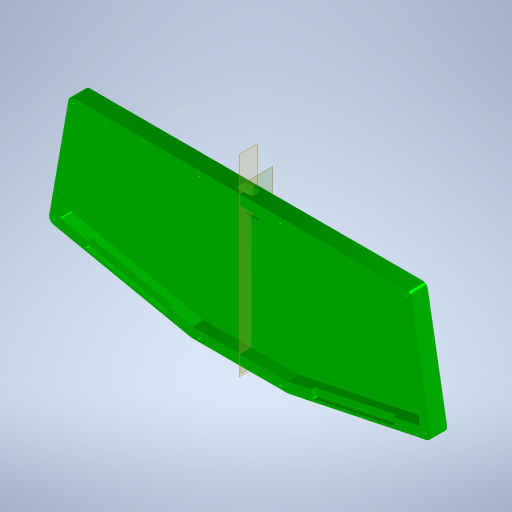
# Autodesk Inventor part: bottom-case
Saved by Autodesk Inventor 2023 (Build 270158000, 158)
## iProperties
Created: 2022-09-09
Part Number: bottom-case
Material: Aluminum 6061-AHC
Document SubType Name: Modeling
Designer: hainguyen
Density: 2.7 g/cm^3
Appearance: Aluminum - Dark
Author: hainguyen
Autodesk Inventor part; units mm, degrees
ref_plane "YZ Plane" through (0, 0, 0) normal (1, 0, 0) x (0, 1, 0)
ref_plane "XZ Plane" through (0, 0, 0) normal (0, 1, 0) x (-1, 0, 0)
ref_plane "XY Plane" through (0, 0, 0) normal (0, 0, 1) x (1, 0, 0)
sketch "Sketch1" plane through (0, 0, 0) normal (0, 0, 1) x (1, 0, 0)
  line L0 (21.6076, -129.4029) -> (96.5033, -129.4029) construction
  line L1 (96.5033, -129.4029) -> (135.6521, -121.1948) construction
  line L2 (-17.5411, -121.1947) -> (21.6076, -129.4029) construction
  line L3 (-68.8789, -30.3383) -> (-82.3292, -106.6218) construction
  line L4 (200.4404, -106.6223) -> (186.9912, -30.3383) construction
  line L5 (121.8455, -29.5119) -> (-68.8789, -29.5119) construction
  line L6 (-69.5723, -28.5119) -> (187.6846, -28.5119)
  line L7 (187.6846, -28.5119) -> (201.7615, -108.3559)
  line L8 (201.7615, -108.3559) -> (96.607, -130.4029)
  line L9 (96.607, -130.4029) -> (21.5039, -130.4029)
  line L10 (21.5039, -130.4029) -> (-83.6503, -108.3555)
  line L11 (-83.6503, -108.3555) -> (-69.5723, -28.5119)
  point P0 (0, 0)
  dimension "d0" = 1
  dimension "d1" = 1
  dimension "d2" = 1
  dimension "d3" = 1
  dimension "d4" = 1
  dimension "d5" = 1
  constraints: 14 end point, 7 parallel, 2 horizontal, 2 other
  measures "d0" distance between parallel lines of L6 L5
  measures "d1" distance between parallel lines of L3 L11
  measures "d2" distance between parallel lines of L2 L10
  measures "d3" distance between parallel lines of L0 L9
  measures "d4" distance between parallel lines of L1 L8
  measures "d5" distance between parallel lines of L4 L7
extrude "Extrusion1" add sketch "Sketch1" along normal blind 17
shell "Shell1" thickness 8 outward yes removed faces 1 at (71.5731, -62.4756, 17)
sketch "Sketch5" plane through (-69.5723, -28.5119, 0) normal (0, 0, 1) x (1, 0, 0)
  line L0 (-14.0781, -79.8436) -> (91.0762, -101.891) projected
  line L1 (91.0762, -101.891) -> (166.1793, -101.891) projected
  line L2 (166.1793, -101.891) -> (271.3337, -79.844) projected
  line L3 (271.3337, -79.844) -> (257.2569, 0) projected
  line L4 (257.2569, 0) -> (0, 0) projected
  line L5 (0, 0) -> (-14.0781, -79.8436) projected
  point P0 (69.5723, 28.5119)
extrude "Extrusion7" add sketch "Sketch5" along normal blind 8
ref_plane "Work Plane1" through (59.0626, 747.1099, -8) normal (-1, 0.0000081, 0) x (0, 0, 1)
sketch "Sketch7" plane through (-76.2851, -20.5119, 17) normal (0, 1, 0) x (1, 0, 0)
  line L0 (131.2466, 4.8) -> (139.4466, 4.8) construction
  line L1 (132.1766, 8.53) -> (138.5266, 8.53) construction
  line L2 (141.8266, 2.8) -> (128.8766, 2.8)
  line L3 (128.8766, 2.8) -> (128.8766, 10.53)
  line L4 (128.8766, 10.53) -> (141.8266, 10.53)
  line L5 (141.8266, 10.53) -> (141.8266, 2.8)
  line L6 (130.8766, 6.67) -> (130.8766, 7.23) construction
  line L7 (139.8266, 7.23) -> (139.8266, 6.67) construction
  point P0 (76.2851, 17)
  point P1 (128.8766, 6.665)
  point P2 (130.8766, 6.95)
  dimension "d25" = 2
  dimension "d26" = 2
  dimension "d27" = 2
  dimension "d28" = 2
  constraints: 8 end point, 2 midpoint, 2 parallel, 1 horizontal, 1 perpendicular
  measures "d25" horizontal distance of point (128.877, 6.665) point (130.877, 6.95)
  measures "d26" distance from line of L5 L7.end
  measures "d27" distance between parallel lines of L1 L4
  measures "d28" distance between parallel lines of L0 L2
extrude "Extrusion9" cut sketch "Sketch7" against normal blind 20
fillet "Fillet2" radius 3 4 edges at (65.5415, -24.5119, 14.2) (65.5415, -30.5119, 6.47) (52.5915, -24.5119, 14.2) (52.5915, -30.5119, 6.47)
sketch "Sketch12" plane through (0, 0, 17) normal (0, 0, 1) x (1, 0, 0)
  line L0 (102.8455, -23.0119) -> (165.8455, -23.0119) construction
  line L1 (121.8455, -29.5119) -> (-67.894, -29.5119) construction
  line L2 (121.8455, -29.5119) -> (-67.894, -29.5119) construction
  line L3 (-47.7327, -23.0102) -> (15.2673, -23.0112) construction
  line L4 (-17.5411, -121.1947) -> (21.6076, -129.4029) construction
  line L5 (-0.2792, -131.4544) -> (-61.9383, -118.5257) construction
  line L6 (180.0496, -118.5277) -> (118.3902, -131.4553) construction
  line L7 (96.5033, -129.4029) -> (135.6521, -121.1948) construction
  line L8 (167.3455, -29.5119) -> (167.3455, -22.5119)
  line L9 (167.3455, -22.5119) -> (101.3455, -22.5119)
  line L10 (101.3455, -22.5119) -> (101.3455, -29.5119)
  line L11 (101.3455, -29.5119) -> (167.3455, -29.5119)
  line L12 (16.7672, -29.5119) -> (16.7672, -22.5119)
  line L13 (16.7672, -22.5119) -> (-49.2328, -22.5119)
  line L14 (16.7672, -29.5119) -> (-49.2328, -29.5119)
  line L15 (96.5033, -129.4029) -> (135.6521, -121.1948) construction
  line L16 (115.5884, -125.4015) -> (117.0248, -132.2525)
  line L17 (117.0248, -132.2525) -> (181.6203, -118.7092)
  line L18 (181.6203, -118.7092) -> (180.1839, -111.8582)
  line L19 (115.5884, -125.4015) -> (180.1839, -111.8582)
  line L20 (-81.5496, -107.7742) -> (-42.0091, -116.0645) construction
  line L21 (2.5226, -125.4014) -> (1.0863, -132.2516)
  line L22 (-63.509, -118.7073) -> (-62.0728, -111.8578)
  line L23 (2.5226, -125.4014) -> (-62.0728, -111.8578)
  line L24 (1.0863, -132.2516) -> (-63.509, -118.7073)
  line L25 (-42.4192, -118.0206) -> (-42.0091, -116.0645) construction
  line L26 (-17.5411, -121.1947) -> (-17.9513, -123.151) construction
  line L27 (136.0625, -123.1523) -> (135.6521, -121.1948) construction
  line L28 (121.8455, -29.5119) -> (121.8455, -27.5119) construction
  line L29 (-3.7328, -27.5109) -> (-3.7328, -29.5109) construction
  line L30 (-28.7328, -29.5105) -> (-28.7328, -27.5105) construction
  line L31 (-49.2328, -22.5119) -> (-49.2328, -29.5119)
  line L32 (160.5305, -118.0223) -> (160.1201, -116.0648) construction
  line L33 (146.8455, -29.5119) -> (146.8455, -27.5119) construction
  point P0 (-49.2327, -26.0119)
  point P1 (-28.7328, -28.5105)
  dimension "d48" = 0.5
  dimension "d50" = 0.5
  dimension "d51" = 20.5
  dimension "d52" = 20.5
  dimension "d53" = 20.5
  dimension "d56" = 0.5
  dimension "d57" = 20.5
  dimension "d58" = 20.5
  dimension "d60" = 20.5
  dimension "d78" = 20.5
  dimension "d80" = 20.5
  constraints: 32 end point, 10 point on line, 7 perpendicular, 3 collinear, 3 parallel, 2 vertical, 1 midpoint
  measures "d48" distance between parallel lines of L17 L6
  measures "d50" distance between parallel lines of L24 L5
  measures "d51" distance between parallel lines of L22 L25
  measures "d52" distance between parallel lines of L21 L26
  measures "d53" distance between parallel lines of L16 L27
  measures "d56" distance between parallel lines of L9 L0
  measures "d57" distance between parallel lines of L10 L28
  measures "d58" distance from line of L29.start L12
  measures "d60" distance from line of L31 point (-28.733, -28.51)
  measures "d78" distance between parallel lines of L18 L32
  measures "d80" distance between parallel lines of L8 L33
extrude "Extrusion13" cut sketch "Sketch12" against normal blind 3
fillet "Fillet4" radius 4 4 edges at (-76.2851, -20.5119, 4.5) (194.3976, -20.5119, 4.5) (210.985, -114.5961, 4.5) (-92.874, -114.5955, 4.5)
fillet "Fillet5" radius 1 12 edges at (101.3455, -22.5119, 15.5) (167.3455, -22.5119, 15.5) (187.6846, -28.5119, 12.5) (-49.2328, -22.5119, 15.5) (16.7672, -22.5119, 15.5) (181.6203, -118.7092, 15.5) (117.0248, -132.2525, 15.5) (1.0863, -132.2516, 15.5) (-63.509, -118.7073, 15.5) (-69.5723, -28.5119, 12.5) (-83.6503, -108.3555, 12.5) (201.7615, -108.3559, 12.5)
sketch "Sketch14" plane through (0, 0, -8) normal (0, 0, -1) x (-1, 0, 0)
  arc A0 (89.083, -115.3904) -> (92.2014, -110.7809) centre (88.2622, -111.4755) ccw projected
  line L0 (76.8679, -23.8173) -> (92.2014, -110.7809) projected
  arc A1 (76.8679, -23.8173) -> (72.9287, -20.5119) centre (72.9287, -24.5119) ccw projected
  line L1 (-191.0411, -20.5119) -> (72.9287, -20.5119) projected
  arc A2 (-191.0411, -20.5119) -> (-194.9804, -23.8174) centre (-191.0411, -24.5119) ccw projected
  line L2 (-210.3125, -110.7815) -> (-194.9804, -23.8174) projected
  arc A3 (-210.3125, -110.7815) -> (-207.194, -115.3909) centre (-206.3732, -111.476) ccw projected
  line L3 (-97.4367, -138.4029) -> (-207.194, -115.3909) projected
  line L4 (-20.6743, -138.4029) -> (-97.4367, -138.4029) projected
  line L5 (89.083, -115.3904) -> (-20.6743, -138.4029) projected
  point P0 (0, 0)
extrude "Extrusion14" cut sketch "Sketch14" against normal blind 12
sketch "Sketch16" plane through (0, 0, 4) normal (0, 0, -1) x (-1, 0, 0)
  point P0 (0, 0)
sketch "Sketch17" plane through (0, 0, 4) normal (0, 0, -1) x (-1, 0, 0)
  arc A0 (89.083, -115.3904) -> (92.2014, -110.7809) centre (88.2622, -111.4755) ccw projected
  line L0 (89.083, -115.3904) -> (-20.6743, -138.4029) projected
  line L1 (-20.6743, -138.4029) -> (-97.4367, -138.4029) projected
  line L2 (-97.4367, -138.4029) -> (-207.194, -115.3909) projected
  arc A1 (-210.3125, -110.7815) -> (-207.194, -115.3909) centre (-206.3732, -111.476) ccw projected
  line L3 (-210.3125, -110.7815) -> (-194.9804, -23.8174) projected
  arc A2 (-191.0411, -20.5119) -> (-194.9804, -23.8174) centre (-191.0411, -24.5119) ccw projected
  line L4 (-191.0411, -20.5119) -> (72.9287, -20.5119) projected
  arc A3 (76.8679, -23.8173) -> (72.9287, -20.5119) centre (72.9287, -24.5119) ccw projected
  line L5 (76.8679, -23.8173) -> (92.2014, -110.7809) projected
  line L6 (-2.3174, -126.3801) -> (-1.2915, -131.2729) projected
  arc A4 (-1.2915, -131.2729) -> (-0.1076, -132.0464) centre (-0.3128, -131.0676) ccw projected
  line L7 (-0.1076, -132.0464) -> (62.5303, -118.9125) projected
  arc A5 (62.5303, -118.9125) -> (63.3038, -117.7286) centre (62.3251, -117.9338) ccw projected
  line L8 (63.3038, -117.7286) -> (62.278, -112.8365) projected
  line L9 (62.278, -112.8365) -> (82.7026, -108.5542) projected
  arc A6 (82.7026, -108.5542) -> (83.4822, -107.4018) centre (82.4974, -107.5755) ccw projected
  line L10 (83.4822, -107.4018) -> (69.718, -29.3383) projected
  arc A7 (69.718, -29.3383) -> (68.7332, -28.5119) centre (68.7332, -29.5119) ccw projected
  line L11 (68.7332, -28.5119) -> (49.2328, -28.5119) projected
  line L12 (49.2328, -28.5119) -> (49.2328, -23.5119) projected
  arc A8 (49.2328, -23.5119) -> (48.2328, -22.5119) centre (48.2328, -23.5119) ccw projected
  line L13 (48.2328, -22.5119) -> (-15.7672, -22.5119) projected
  arc A9 (-15.7672, -22.5119) -> (-16.7672, -23.5119) centre (-15.7672, -23.5119) ccw projected
  line L14 (-16.7672, -23.5119) -> (-16.7672, -28.5119) projected
  line L15 (-16.7672, -28.5119) -> (-101.3455, -28.5119) projected
  line L16 (-101.3455, -28.5119) -> (-101.3455, -23.5119) projected
  arc A10 (-101.3455, -23.5119) -> (-102.3455, -22.5119) centre (-102.3455, -23.5119) ccw projected
  line L17 (-102.3455, -22.5119) -> (-166.3455, -22.5119) projected
  arc A11 (-166.3455, -22.5119) -> (-167.3455, -23.5119) centre (-166.3455, -23.5119) ccw projected
  line L18 (-167.3455, -23.5119) -> (-167.3455, -28.5119) projected
  line L19 (-167.3455, -28.5119) -> (-186.8455, -28.5119) projected
  arc A12 (-186.8455, -28.5119) -> (-187.8303, -29.3383) centre (-186.8455, -29.5119) ccw projected
  line L20 (-187.8303, -29.3383) -> (-201.5933, -107.4023) projected
  arc A13 (-201.5933, -107.4023) -> (-200.8137, -108.5546) centre (-200.6085, -107.5759) ccw projected
  line L21 (-200.8137, -108.5546) -> (-180.3891, -112.8369) projected
  line L22 (-180.3891, -112.8369) -> (-181.4151, -117.7305) projected
  arc A14 (-181.4151, -117.7305) -> (-180.6416, -118.9145) centre (-180.4364, -117.9357) ccw projected
  line L23 (-180.6416, -118.9145) -> (-118.0035, -132.0473) projected
  arc A15 (-118.0035, -132.0473) -> (-116.8196, -131.2738) centre (-117.7983, -131.0686) ccw projected
  line L24 (-116.8196, -131.2738) -> (-115.7936, -126.3802) projected
  line L25 (-115.7936, -126.3802) -> (-96.607, -130.4029) projected
  line L26 (-96.607, -130.4029) -> (-21.5039, -130.4029) projected
  line L27 (-21.5039, -130.4029) -> (-2.3174, -126.3801) projected
  circle A16 centre (-191.0411, -24.5119) radius 1.7396
  circle A17 centre (-206.3732, -111.476) radius 1.3455
  circle A18 centre (-91.1144, -135.6415) radius 1.736
  circle A19 centre (-91.1144, -24.5119) radius 2.0059
  line L28 (-91.1144, -24.5119) -> (-91.1144, -135.6415)
  line L29 (-91.1144, -135.6415) -> (-206.3732, -111.476) construction
  line L30 (-191.0411, -24.5119) -> (-91.1144, -24.5119) construction
  line L31 (-191.0411, -24.5119) -> (-206.3732, -111.476) construction
  line L32 (-59.0568, 27.6823) -> (-59.0553, -166.0852) projected
  circle A20 centre (72.9283, -24.5098) radius 1.7396
  circle A21 centre (88.2618, -111.4736) radius 1.3455
  circle A22 centre (-26.9966, -135.6409) radius 1.736
  circle A23 centre (-26.9984, -24.5114) radius 2.0059
  point P0 (0, 0)
  dimension "d83" = 64.116
  constraints: 8 centre point, 8 end point, 4 symmetric about line, 2 coincident, 2 parallel, 1 vertical, 4 other
  measures "d83" distance of A23.centre L28.start
ref_plane "Work Plane3" through (59.0626, 747.1099, 17) normal (1, -0.0000081, 0) x (0, 0, -1)
hole "Hole2" at (191.0411, -24.5119, 4) at (206.3732, -111.476, 4) at (91.1144, -135.6415, 4) at (91.1144, -24.5119, 4) at (26.9984, -24.5114, 4) at (26.9966, -135.6409, 4) at (-88.2622, -111.4755, 4) at (-72.9287, -24.5119, 4) direction (0, 0, 1) diameter 2 end through all counterbore diameter 4 counterbore depth 8
equation "\"d1\" = d0"
equation "\"d2\" = d0"
equation "\"d3\" = d0"
equation "\"d4\" = d0"
equation "\"d5\" = d0"
body "Solid1"
